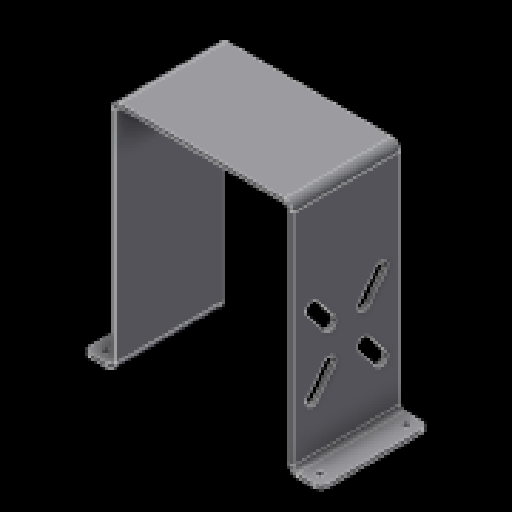
# Autodesk Inventor part: BatteryMount
Saved by Autodesk Inventor 2025.2 (Build 292293000, 293)
## iProperties
Created: 2025-11-21
Part Number: BatteryMount
Material: Generic
Document SubType Name: Sheet Metal
Designer: valer
Density: 1 g/cm^3
Sheet Metal Rule: Default
Appearance: Default
Author: valer
Autodesk Inventor part; units mm, degrees
ref_plane "YZ Plane" through (0, 0, 0) normal (1, 0, 0) x (0, 1, 0)
ref_plane "XZ Plane" through (0, 0, 0) normal (0, 1, 0) x (-1, 0, 0)
ref_plane "XY Plane" through (0, 0, 0) normal (0, 0, 1) x (1, 0, 0)
sketch "Base" plane through (0, 0, 0) normal (0, 0, 1) x (1, 0, 0)
  line L0 (161.5, 0) -> (161.5, 216)
  line L1 (161.5, 216) -> (0, 216)
  line L2 (0, 216) -> (0, 0)
  line L3 (0, 208.5) -> (0, 14)
  line L4 (-30, -5) -> (-30, 0) construction
  line L5 (161.5, 0) -> (191.5, 0)
  line L6 (0, 0) -> (-30, 0)
  line L7 (0, 0) -> (161.5, 0) construction
  line L8 (80.75, 0) -> (80.75, 216) construction
  dimension "d1" = 30
  dimension "d4" = 161.5
  dimension "d5" = 216
  measures "d1" distance of L2.end L6.end
  measures "d4" distance of L0.end L1.end
  measures "d5" distance of L0.start L0.end
contour flange "BaseFeature" sketch "Base" thickness 4 bend radius 4 width 100 along (0, 0, 1) mid plane no both sides no wall seen from (176.5, 0, 0) lies toward (0, 1, 0) curves L5 L0 L1 L2 L6
bend "Bend1"
corner "Corner1"
sketch "MountHoles" plane through (191.5, 4, 100) normal (0, 1, 0) x (1, 0, 0)
  line L0 (0, 100) -> (-22, 100) projected
  line L1 (-11, 100) -> (-11, 0) construction
  line L2 (0, 0) -> (-22, 0) projected
  line L3 (-34, 100) -> (-187.5, 100) projected
  line L4 (-110.75, 100) -> (-110.75, 0) construction
  line L5 (-34, 0) -> (-187.5, 0) projected
  circle A0 centre (-11, 90) radius 3
  line L6 (0, 100) -> (0, 0) projected
  line L7 (0, 50) -> (-11, 50) construction
  circle A1 centre (-11, 10) radius 3
  circle A2 centre (-210.5, 90) radius 3
  circle A3 centre (-210.5, 10) radius 3
  point P0 (-191.5, 100)
  dimension "d17" = 6
  dimension "d18" = 10
  constraints: 6 end point, 6 midpoint, 4 centre point, 3 symmetric about line, 1 point on line, 3 other
  measures "d17" diameter of A0
  measures "d18" distance from line of L0 A0.centre
extrude "MountHolesFeature" cut sketch "MountHoles" against normal blind 4
fillet "FilletsFeature" radius 6 4 edges at (191.5, 2, 0) (191.5, 2, 100) (-30, 2, 0) (-30, 2, 100)
sketch "Slots" plane through (165.5, 8, 100) normal (1, 0, 0) x (0, 0, -1)
  line L0 (82, 45) -> (66, 65.4791) construction
  line L1 (86.7281, 48.694) -> (70.7281, 69.173)
  line L2 (61.2719, 61.7851) -> (77.2719, 41.306)
  arc A0 (77.2719, 41.306) -> (86.7281, 48.694) centre (82, 45) ccw
  arc A1 (70.7281, 69.173) -> (61.2719, 61.7851) centre (66, 65.4791) ccw
  line L3 (94, -4) -> (6, -4) projected
  line L4 (50, -4) -> (50, 204) construction
  line L5 (100, 204) -> (0, 204) projected
  line L6 (13.2719, 48.694) -> (29.2719, 69.173)
  line L7 (38.7281, 61.7851) -> (22.7281, 41.306)
  arc A2 (13.2719, 48.694) -> (22.7281, 41.306) centre (18, 45) ccw
  arc A3 (38.7281, 61.7851) -> (29.2719, 69.173) centre (34, 65.4791) ccw
  line L8 (100, 0) -> (100, 204) projected
  line L9 (0, 0) -> (100, 0) projected
  line L10 (100, 81.4791) -> (0, 81.4791) construction
  line L11 (0, 0) -> (0, 204) projected
  line L12 (86.7281, 114.2642) -> (70.7281, 93.7851)
  line L13 (61.2719, 101.173) -> (77.2719, 121.6521)
  arc A4 (86.7281, 114.2642) -> (77.2719, 121.6521) centre (82, 117.9581) ccw
  arc A5 (61.2719, 101.173) -> (70.7281, 93.7851) centre (66, 97.4791) ccw
  arc A6 (22.7281, 121.6521) -> (13.2719, 114.2642) centre (18, 117.9581) ccw
  line L14 (38.7281, 101.173) -> (22.7281, 121.6521)
  line L15 (13.2719, 114.2642) -> (29.2719, 93.7851)
  arc A7 (29.2719, 93.7851) -> (38.7281, 101.173) centre (34, 97.4791) ccw
  point P0 (100, -8)
  point P1 (74, 55.2395)
  dimension "d22" = 6
  dimension "d23" = 34
  dimension "d24" = 18
  dimension "d25" = 38
  dimension "d26" = 45
  dimension "d27" = 16
  constraints: 24 end point, 18 symmetric about line, 16 point on circle, 8 centre point, 4 tangent, 3 midpoint, 2 point on line, 1 horizontal, 1 parallel, 6 other
  measures "d22" radius of A0
  measures "d23" distance from line of L8 L0.end
  measures "d24" distance from line of L8 L0.start
  measures "d25" angle of L4 L0
  measures "d26" distance from line of L9 L0.start
  measures "d27" distance from line of L0.end L10
extrude "SlotsFeature" cut sketch "Slots" against normal blind 4 contours A0 L2 A1 L1 | L6 A3 L7 A2 | L12 A5 L13 A4 | L14 A7 L15 A6
equation "\"d19\" = Thickness"
equation "\"d28\" = Thickness"
equation "\"d6\" = Thickness"
equation "\"d7\" = BendReliefWidth"
equation "\"d8\" = BendReliefDepth"
equation "\"d9\" = MinimumRemnant"
equation "\"d10\" = TransitionRadius"
equation "\"d12\" = BendRadius"
equation "\"d14\" = CornerReliefSize"
equation "\"d15\" = GapSize"
equation "\"d16\" = JacobiRadiusSize"
equation "\"BendRadius\" = Thickness"
equation "\"BendReliefWidth\" = Thickness"
equation "\"BendReliefDepth\" = 0.5 * Thickness"
equation "\"CornerReliefSize\" = 4 * Thickness"
equation "\"MinimumRemnant\" = 2 * Thickness"
equation "\"TransitionRadius\" = BendRadius"
equation "\"JacobiRadiusSize\" = BendRadius"
equation "\"GapSize\" = Thickness"
equation "\"Thickness\" = 4"
body "Solid1"
